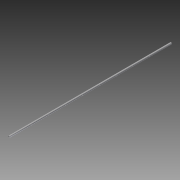
# Autodesk Inventor part: GE-13029
Saved by Autodesk Inventor 2013 (Build 170138000, 138)
## iProperties
Created: 2013-01-03
Part Number: GE-13029
Material: Steel
Document SubType Name: Modeling
Designer: Phillip
Density: 1 g/cm^3
Author: Phillip
Autodesk Inventor part; units mm, degrees
ref_plane "YZ Plane" through (0, 0, 0) normal (1, 0, 0) x (0, 1, 0)
ref_plane "XY Plane" through (0, 0, 0) normal (0, 0, 1) x (1, 0, 0)
sketch "Sketch1" plane through (0, 0, 0) normal (0, 0, 1) x (1, 0, 0)
  circle A0 centre (0, 0) radius 8.5725
  circle A1 centre (0, 0) radius 6.2611
  dimension "d0" = 17.145
  dimension "d2" = 2.3114
  constraints: 2 centre point, 2 coincident
  measures "d0" diameter of A0
  measures "d2" radial gap between concentric circles of A0 A1
extrude "Extrusion1" add sketch "Sketch1" against normal blind 1587.5
ref_plane "Work Plane1" through (0, 8.5725, 0) normal (0, 1, 0) x (-1, 0, 0)
sketch "Sketch2" plane through (0, 8.5725, 0) normal (0, 1, 0) x (-1, 0, 0)
  line L0 (-8.5725, 0) -> (8.5725, 0) projected
  point P0 (0, 0)
  point P1 (0, -215.9)
  point P2 (0, -381)
  point P3 (0, -546.1)
  point P4 (0, -711.2)
  point P5 (0, 0)
  point P6 (0, -876.3)
  point P7 (0, -1041.4)
  point P8 (0, -1206.5)
  point P9 (0, -1371.6)
  dimension "d5" = 215.9
  dimension "d6" = 381
  dimension "d7" = 546.1
  dimension "d8" = 711.2
  dimension "d16" = 876.3
  dimension "d17" = 1041.4
  dimension "d18" = 1206.5
  dimension "d19" = 1371.6
  constraints: 8 vertical alignment, 1 midpoint
  measures "d5" distance from line of point (0, -215.9) L0
  measures "d6" distance from line of point (0, -381) L0
  measures "d7" distance from line of point (0, -546.1) L0
  measures "d8" distance from line of point (0, -711.2) L0
  measures "d16" distance from line of L0 point (0, -876.3)
  measures "d17" distance from line of L0 point (0, -1041.4)
  measures "d18" distance from line of L0 point (0, -1206.5)
  measures "d19" distance from line of L0 point (0, -1371.6)
hole "Hole1" at (0, 8.5725, -215.9) at (0, 8.5725, -381) at (0, 8.5725, -546.1) at (0, 8.5725, -711.2) at (0, 8.5725, -876.3) at (0, 8.5725, -1041.4) at (0, 8.5725, -1206.5) at (0, 8.5725, -1371.6) direction (0, -1, 0) diameter 5.08 end through all
body "Solid1"
